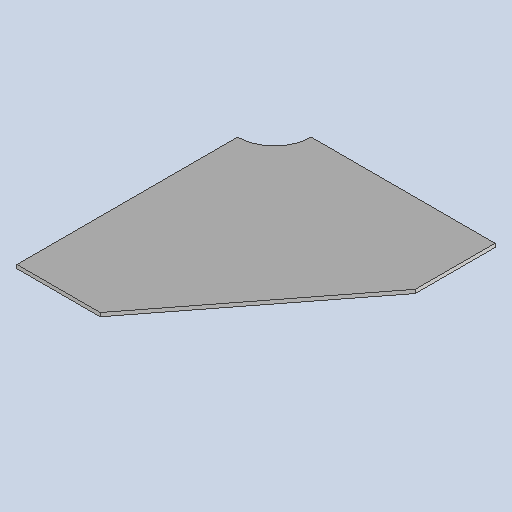
# Autodesk Inventor part: TRM 034 motor pillar
Saved by Autodesk Inventor 2025 (Build 290162010, 162A)
## iProperties
Created: 2024-08-07
Part Number: TRM 034 motor pillar
Material: AISI 304
Document SubType Name: Sheet Metal
Designer: user
Stock Number: ТРМ 023 лицо успокоитель
Density: 8.02768 g/cm^3
Flat Pattern Width: 12 cm
Flat Pattern Length: 14 cm
Flat Pattern Area: 168 cm^2
Sheet Metal Rule: AISI304 2mm Die16
Sheet Metal Width: 120.000 mm
Sheet Metal Length: 140.000 mm
Sheet Metal Area: 16800.000 mm^2
Appearance: Default
Mass: 206.703 g
Surface Area: 266.732 cm^2
Volume: 25.7488 cm^3
Author: pokla
Autodesk Inventor part; units mm, degrees
ref_plane "YZ Plane" through (0, 0, 0) normal (1, 0, 0) x (0, 1, 0)
ref_plane "XZ Plane" through (0, 0, 0) normal (0, 1, 0) x (-1, 0, 0)
ref_plane "XY Plane" through (0, 0, 0) normal (0, 0, 1) x (1, 0, 0)
sketch "Sketch1" plane through (0, 0, 0) normal (0, 0, 1) x (1, 0, 0)
  line L0 (-60, -70) -> (60, -70)
  line L1 (60, -70) -> (60, 70)
  line L2 (60, 70) -> (-60, 70)
  line L3 (-60, 70) -> (-60, -70)
  line L4 (-60, -70) -> (60, 70) construction
  line L5 (60, -70) -> (-60, 70) construction
  line L6 (-60, 0) -> (60, 0) construction
  circle A0 centre (-60, 70) radius 20
  line L7 (60, 26.6315) -> (-14.7466, -70)
  point P0 (0, 0)
  point P1 (0, 0)
  point P2 (-40, 70)
  point P3 (-60, 50)
  dimension "d0" = 120
  dimension "d1" = 140
  dimension "d16" = 40
  measures "d0" distance of L2.end L1.end
  measures "d1" distance of L1.end L0.end
  measures "d16" diameter of A0
extrude "Plate1" add sketch "Sketch1" along normal blind 2 contours L3 A0 L2 L1 L7 L0
sketch "Sketch2" plane through (0, 0, 0) normal (0, 0, -1) x (-1, 0, 0)
  line L0 (-40, 50) -> (160, 50) construction
  line L1 (160, 50) -> (160, 30) construction
  line L2 (160, 30) -> (-40, 30) construction
  line L3 (-40, 30) -> (-40, 50) construction
  line L4 (-60, 70) -> (40, 70) projected
  line L5 (-60, 26.6315) -> (-60, 70) projected
  point P0 (0, 0)
  point P1 (-48, 100)
  point P2 (60, 70)
  point P3 (-60, -70)
  point P4 (-50, 98)
  dimension "d6" = 200
  dimension "d9" = 20
  dimension "d10" = 20
  dimension "d11" = 20
  constraints: 4 other
  measures "d6" distance of L0.start L0.end
  measures "d9" distance of L0.end L1.end
  measures "d11" length of L3
mark "Mark1"
equation "\"d2\" = Thickness"
equation "\"BendReliefWidth\" = Thickness"
equation "\"BendReliefDepth\" = 0.5 * Thickness"
equation "\"CornerReliefSize\" = 4 * Thickness"
equation "\"MinimumRemnant\" = 2 * Thickness"
equation "\"TransitionRadius\" = BendRadius"
equation "\"JacobiRadiusSize\" = BendRadius"
equation "\"GapSize\" = Thickness"
equation "\"Thickness\" = 2"
equation "\"BendRadius\" = 2.75"
body "Solid1"
